Autodesk Fusion 360 part; units mm, degrees
(part 12 of 25)
  arc A2061 (18.3325, 43.4756) -> (18.0149, 43.4756) centre (18.1737, 43.4756) ccw
  arc A2062 (27.9971, 41.2945) -> (28.3146, 41.2945) centre (28.1559, 41.2945) ccw
  arc A2063 (24.9949, 41.4591) -> (24.9949, 41.7766) centre (24.9949, 41.6179) ccw
  arc A2064 (4.8319, 35.4266) -> (4.8319, 35.1091) centre (4.8319, 35.2678) ccw
  arc A2065 (18.3765, 38.645) -> (18.6594, 38.5008) centre (18.5179, 38.5729) ccw
  line L663 (18.8179, 41.8997) -> (18.3999, 41.4817)
  arc A2066 (18.7474, 38.6736) -> (18.4645, 38.8177) centre (18.606, 38.7457) ccw
  line L664 (18.458, 38.3885) -> (18.4277, 38.197)
  line L665 (21.7972, 41.91) -> (21.8221, 41.9203)
  arc A2067 (22.1278, 43.9094) -> (22.3523, 44.1339) centre (22.2401, 44.0217) ccw
  arc A2068 (27.2855, 43.2371) -> (27.2855, 43.5546) centre (27.2855, 43.3959) ccw
  arc A2069 (18.5865, 38.197) -> (18.269, 38.197) centre (18.4277, 38.197) ccw
  arc A2070 (27.3977, 43.5082) -> (27.1732, 43.2836) centre (27.2855, 43.3959) ccw
  arc A2071 (18.5122, 42.4506) -> (18.2877, 42.226) centre (18.4, 42.3383) ccw
  line L666 (18.4277, 38.197) -> (18.4277, 38.1)
  line L667 (21.8221, 41.9203) -> (22.2401, 42.3383)
  arc A2072 (19.1107, 39.0872) -> (19.2322, 39.3805) centre (19.1715, 39.2339) ccw
  line L668 (26.0545, 43.3959) -> (25.1841, 42.5255)
  arc A2073 (18.3204, 42.9452) -> (18.027, 42.8237) centre (18.1737, 42.8845) ccw
  arc A2074 (24.8827, 41.7302) -> (25.1072, 41.5056) centre (24.9949, 41.6179) ccw
  line L669 (18.8571, 39.0396) -> (18.72, 38.9025)
  arc A2075 (18.8786, 42.067) -> (18.7572, 41.7736) centre (18.8179, 41.9203) ccw
  line L670 (28.1559, 41.2945) -> (28.1559, 42.5255)
  line L671 (19.364, 44.6659) -> (18.8179, 44.4397)
  arc A2076 (26.0545, 43.5546) -> (26.0545, 43.2371) centre (26.0545, 43.3959) ccw
  line L672 (22.2401, 42.3383) -> (22.4663, 42.8844)
  arc A2077 (22.625, 43.4756) -> (22.3075, 43.4756) centre (22.4663, 43.4756) ccw
  arc A2078 (26.1668, 43.2836) -> (25.9423, 43.5082) centre (26.0545, 43.3959) ccw
  arc A2079 (18.2877, 44.1339) -> (18.5122, 43.9094) centre (18.4, 44.0217) ccw
  line L673 (18.518, 38.5729) -> (18.458, 38.3885)
  line L674 (18.1737, 40.9356) -> (18.1737, 40.3444)
  arc A2080 (21.8579, 42.0567) -> (21.7364, 41.7633) centre (21.7972, 41.91) ccw
  arc A2081 (18.269, 38.1) -> (18.5865, 38.1) centre (18.4277, 38.1) ccw
  line L675 (22.4663, 43.4756) -> (22.2401, 44.0217)
  arc A2082 (25.2964, 41.6948) -> (25.0718, 41.9193) centre (25.1841, 41.807) ccw
  arc A2083 (18.027, 43.5363) -> (18.3204, 43.4148) centre (18.1737, 43.4755) ccw
  arc A2084 (18.027, 40.9963) -> (18.3204, 40.8748) centre (18.1737, 40.9356) ccw
  arc A2085 (18.4776, 38.839) -> (18.7344, 38.6523) centre (18.606, 38.7456) ccw
  arc A2086 (18.3071, 38.4375) -> (18.609, 38.3394) centre (18.4581, 38.3885) ccw
  arc A2087 (18.2532, 42.2776) -> (18.5466, 42.3991) centre (18.3999, 42.3383) ccw
  line L676 (21.4533, 36.9584) -> (21.6261, 37.0464)
  arc A2088 (18.2709, 38.2218) -> (18.5845, 38.1721) centre (18.4277, 38.197) ccw
  arc A2089 (19.4248, 44.5192) -> (19.3033, 44.8126) centre (19.364, 44.6659) ccw
  line L677 (19.0139, 39.1536) -> (18.8571, 39.0396)
  arc A2090 (18.6689, 38.5238) -> (18.367, 38.6219) centre (18.518, 38.5729) ccw
  arc A2091 (18.7821, 41.7633) -> (18.9035, 42.0567) centre (18.8428, 41.91) ccw
  arc A2092 (18.3204, 40.4052) -> (18.027, 40.2837) centre (18.1737, 40.3444) ccw
  arc A2093 (19.2435, 39.0924) -> (19.0994, 39.3753) centre (19.1715, 39.2339) ccw
  arc A2094 (18.9302, 41.7874) -> (18.7056, 42.0119) centre (18.8179, 41.8997) ccw
  line L678 (18.606, 38.7457) -> (18.518, 38.5729)
  line L679 (18.8179, 39.3803) -> (19.1715, 39.2339)
  arc A2095 (18.7638, 39.1681) -> (18.9504, 38.9112) centre (18.8571, 39.0397) ccw
  arc A2096 (18.9036, 41.7633) -> (18.7821, 42.0567) centre (18.8429, 41.91) ccw
  line L680 (19.1715, 39.2339) -> (19.0139, 39.1536)
  arc A2097 (18.3325, 40.9356) -> (18.0149, 40.9356) centre (18.1737, 40.9356) ccw
  arc A2098 (18.5466, 43.9609) -> (18.2532, 44.0824) centre (18.3999, 44.0217) ccw
  line L681 (18.3999, 42.3383) -> (18.8179, 41.9203)
  line L682 (18.1737, 40.3444) -> (18.3999, 39.7983)
  arc A2099 (18.7056, 41.8081) -> (18.9302, 42.0326) centre (18.8179, 41.9203) ccw
  arc A2100 (18.0149, 40.3444) -> (18.3325, 40.3444) centre (18.1737, 40.3444) ccw
  line L683 (18.3999, 44.0217) -> (18.1737, 43.4756)
  line L684 (18.3999, 39.7983) -> (18.8179, 39.3803)
  arc A2101 (18.9419, 39.2951) -> (19.086, 39.0122) centre (19.014, 39.1537) ccw
  arc A2102 (19.1073, 39.0252) -> (18.9206, 39.282) centre (19.014, 39.1536) ccw
  arc A2103 (18.8484, 38.8092) -> (18.5915, 38.9958) centre (18.72, 38.9025) ccw
  line L685 (18.1737, 43.4756) -> (18.1737, 42.8844)
  arc A2104 (18.7056, 39.2681) -> (18.9302, 39.4926) centre (18.8179, 39.3803) ccw
  arc A2105 (18.2532, 39.7376) -> (18.5466, 39.8591) centre (18.3999, 39.7984) ccw
  line L686 (18.8179, 41.9203) -> (18.8428, 41.91)
  line L687 (18.72, 38.9025) -> (18.606, 38.7457)
  line L688 (18.3999, 41.4817) -> (18.1737, 40.9356)
  line L689 (18.8428, 41.91) -> (18.8179, 41.8997)
  line L690 (18.8179, 44.4397) -> (18.3999, 44.0217)
  arc A2106 (21.2937, 36.7416) -> (21.244, 37.0552) centre (21.2689, 36.8984) ccw
  arc A2107 (18.7572, 42.0463) -> (18.8787, 41.753) centre (18.818, 41.8997) ccw
  arc A2108 (18.8787, 39.527) -> (18.7572, 39.2336) centre (18.8179, 39.3803) ccw
  arc A2109 (18.9693, 38.9274) -> (18.7448, 39.1519) centre (18.8571, 39.0397) ccw
  arc A2110 (18.0149, 42.8844) -> (18.3325, 42.8844) centre (18.1737, 42.8844) ccw
  arc A2111 (18.5122, 39.9106) -> (18.2877, 39.686) centre (18.4, 39.7983) ccw
  arc A2112 (18.6077, 39.0148) -> (18.8322, 38.7903) centre (18.72, 38.9026) ccw
  arc A2113 (18.6148, 38.3636) -> (18.3012, 38.4133) centre (18.458, 38.3884) ccw
  line L691 (18.1737, 42.8844) -> (18.3999, 42.3383)
  arc A2114 (18.2877, 41.5939) -> (18.5122, 41.3694) centre (18.4, 41.4817) ccw
  arc A2115 (33.9077, 4.9657) -> (34.1322, 4.7412) centre (34.02, 4.8535) ccw
  arc A2116 (21.1166, 13.6842) -> (21.1166, 14.0017) centre (21.1166, 13.843) ccw
  arc A2117 (13.9383, 12.0328) -> (13.6208, 12.0328) centre (13.7796, 12.0328) ccw
  line L692 (33.3711, 4.5847) -> (34.02, 4.8535)
  arc A2118 (13.8918, 10.9141) -> (13.6672, 10.6896) centre (13.7795, 10.8018) ccw
  arc A2119 (34.4478, 4.7412) -> (34.6723, 4.9657) centre (34.5601, 4.8535) ccw
  arc A2120 (35.2089, 4.7435) -> (35.2089, 4.426) centre (35.2089, 4.5848) ccw
  arc A2121 (16.3207, 14.0017) -> (16.3207, 13.6842) centre (16.3207, 13.843) ccw
  line L693 (31.6665, 5.207) -> (32.02, 4.8535)
  arc A2122 (17.1338, 11.4447) -> (16.9093, 11.6693) centre (17.0216, 11.557) ccw
  line L694 (22.559, 12.0525) -> (22.86, 12.3536)
  line L695 (16.3207, 13.843) -> (15.9006, 13.669)
  arc A2123 (16.639, 11.399) -> (16.8636, 11.1745) centre (16.7513, 11.2867) ccw
  line L696 (15.8809, 9.9314) -> (16.7513, 10.8018)
  arc A2124 (21.8174, 11.3983) -> (21.8174, 11.7157) centre (21.8174, 11.557) ccw
  arc A2125 (15.7686, 10.0437) -> (15.9931, 9.8191) centre (15.8808, 9.9314) ccw
  line L697 (34.29, 5.1235) -> (34.56, 4.8535)
  arc A2126 (22.9723, 12.4658) -> (22.7477, 12.2413) centre (22.86, 12.3536) ccw
  arc A2127 (16.8636, 10.6896) -> (16.639, 10.9141) centre (16.7513, 10.8019) ccw
  arc A2128 (22.2982, 11.5843) -> (22.1767, 11.8777) centre (22.2375, 11.731) ccw
  line L698 (13.7795, 10.8018) -> (14.6499, 9.9314)
  arc A2129 (35.1481, 4.438) -> (35.2696, 4.7314) centre (35.2088, 4.5847) ccw
  line L699 (16.7513, 11.2868) -> (17.0215, 11.557)
  arc A2130 (31.6665, 5.0482) -> (31.6665, 5.3658) centre (31.6665, 5.207) ccw
  line L700 (14.6499, 9.9314) -> (15.8809, 9.9314)
  arc A2131 (32.6081, 4.438) -> (32.7296, 4.7314) centre (32.6689, 4.5847) ccw
  line L701 (16.7513, 10.8018) -> (16.7513, 11.2868)
  arc A2132 (15.8809, 9.7727) -> (15.8809, 10.0901) centre (15.8809, 9.9314) ccw
  arc A2133 (21.7566, 11.7037) -> (21.8781, 11.4103) centre (21.8173, 11.557) ccw
  arc A2134 (16.91, 11.2868) -> (16.5925, 11.2868) centre (16.7513, 11.2868) ccw
  line L702 (29.8325, 5.381) -> (30.2526, 5.207)
  line L703 (35.2089, 4.5847) -> (35.9111, 4.5847)
  arc A2135 (29.7203, 5.2688) -> (29.9448, 5.4933) centre (29.8326, 5.3811) ccw
  arc A2136 (34.0807, 4.7068) -> (33.9592, 5.0001) centre (34.02, 4.8535) ccw
  arc A2137 (30.1919, 5.0603) -> (30.3134, 5.3537) centre (30.2527, 5.207) ccw
  line L704 (30.2526, 5.207) -> (31.6665, 5.207)
  arc A2138 (14.5377, 9.8191) -> (14.7622, 10.0437) centre (14.65, 9.9314) ccw
  arc A2139 (16.5925, 10.8018) -> (16.91, 10.8018) centre (16.7513, 10.8018) ccw
  line L705 (21.8174, 11.557) -> (22.2375, 11.731)
  arc A2140 (35.8504, 4.7314) -> (35.9719, 4.438) centre (35.9112, 4.5847) ccw
  arc A2141 (30.2526, 5.3658) -> (30.2526, 5.0482) centre (30.2526, 5.207) ccw
  arc A2142 (22.1252, 11.8433) -> (22.3497, 11.6188) centre (22.2375, 11.731) ccw
  line L706 (32.02, 4.8535) -> (32.6689, 4.5847)
  line L707 (34.56, 4.8535) -> (35.2089, 4.5847)
  arc A2143 (31.9078, 4.7412) -> (32.1323, 4.9657) centre (32.0201, 4.8535) ccw
  arc A2144 (29.8933, 5.5277) -> (29.7718, 5.2343) centre (29.8325, 5.381) ccw
  arc A2145 (36.6207, 4.7068) -> (36.4992, 5.0001) centre (36.56, 4.8534) ccw
  line L708 (22.2375, 11.731) -> (22.559, 12.0525)
  arc A2146 (21.6047, 15.0442) -> (21.8293, 15.2687) centre (21.717, 15.1564) ccw
  arc A2147 (34.4023, 5.0112) -> (34.1777, 5.2357) centre (34.29, 5.1235) ccw
  arc A2148 (32.0808, 5.0001) -> (31.9593, 4.7068) centre (32.0201, 4.8534) ccw
  arc A2149 (31.7787, 5.3193) -> (31.5542, 5.0947) centre (31.6665, 5.207) ccw
  arc A2150 (34.4023, 5.2357) -> (34.1777, 5.0112) centre (34.29, 5.1234) ccw
  line L709 (35.9111, 4.5847) -> (36.56, 4.8535)
  arc A2151 (34.6208, 5.0001) -> (34.4993, 4.7068) centre (34.5601, 4.8535) ccw
  arc A2152 (22.9723, 12.2413) -> (22.7477, 12.4658) centre (22.86, 12.3536) ccw
  line L710 (17.0215, 11.557) -> (21.8174, 11.557)
  arc A2153 (22.4467, 12.1648) -> (22.6712, 11.9403) centre (22.5589, 12.0526) ccw
  arc A2154 (14.6499, 10.0901) -> (14.6499, 9.7727) centre (14.6499, 9.9314) ccw
  line L711 (32.6689, 4.5847) -> (33.3711, 4.5847)
  arc A2155 (35.9111, 4.426) -> (35.9111, 4.7435) centre (35.9111, 4.5848) ccw
  arc A2156 (22.6712, 11.9403) -> (22.4467, 12.1648) centre (22.5589, 12.0526) ccw
  arc A2157 (17.0215, 11.7157) -> (17.0215, 11.3983) centre (17.0215, 11.557) ccw
  line L712 (22.86, 12.3536) -> (29.8325, 5.381)
  arc A2158 (38.1941, 4.9955) -> (38.2438, 4.6819) centre (38.2189, 4.8387) ccw
  line L713 (37.7461, 4.8759) -> (37.9811, 4.8387)
  arc A2159 (38.2588, 6.35) -> (37.9413, 6.35) centre (38.1, 6.35) ccw
  arc A2160 (39.5995, 5.4777) -> (39.375, 5.2532) centre (39.4873, 5.3655) ccw
  arc A2161 (37.5689, 5.1004) -> (37.4708, 4.7984) centre (37.5199, 4.9494) ccw
  arc A2162 (38.6081, 5.0909) -> (38.7522, 4.808) centre (38.6802, 4.9495) ccw
  arc A2163 (37.9412, 4.8387) -> (38.2587, 4.8387) centre (38.0999, 4.8387) ccw
  line L714 (39.4872, 5.3655) -> (39.6555, 5.1972)
  arc A2164 (39.365, 5.2532) -> (39.1405, 5.4777) centre (39.2528, 5.3655) ccw
  line L715 (34.02, 4.8535) -> (34.29, 5.1235)
  arc A2165 (33.3104, 4.7314) -> (33.4319, 4.438) centre (33.3712, 4.5847) ccw
  arc A2166 (38.2189, 4.6799) -> (38.2189, 4.9975) centre (38.2189, 4.8387) ccw
  line L716 (37.1155, 5.1972) -> (37.3079, 5.0574)
  arc A2167 (39.5432, 5.085) -> (39.7677, 5.3095) centre (39.6555, 5.1973) ccw
  arc A2168 (37.9562, 4.6819) -> (38.0059, 4.9955) centre (37.9811, 4.8387) ccw
  arc A2169 (38.1, 6.5087) -> (38.1, 6.1912) centre (38.1, 6.35) ccw
  line L717 (37.9811, 4.8387) -> (38.1, 4.8387)
  arc A2170 (39.9878, 4.808) -> (40.1319, 5.0909) centre (40.0599, 4.9494) ccw
  line L718 (38.1, 4.8387) -> (38.2189, 4.8387)
  line L719 (39.6555, 5.1972) -> (39.8479, 5.0574)
  line L720 (38.1, 4.8387) -> (38.1, 6.35)
  line L721 (37.0096, 5.3031) -> (37.1155, 5.1972)
  line L722 (39.37, 5.5268) -> (39.4872, 5.3655)
  arc A2171 (38.4048, 5.0269) -> (38.503, 4.7249) centre (38.4539, 4.8759) ccw
  arc A2172 (38.9642, 4.916) -> (38.82, 5.1989) centre (38.8921, 5.0575) ccw
  line L723 (38.6801, 4.9494) -> (38.8921, 5.0574)
  line L724 (38.8921, 5.0574) -> (39.0845, 5.1972)
  arc A2173 (39.7488, 5.3257) -> (39.5621, 5.0688) centre (39.6555, 5.1973) ccw
  arc A2174 (37.7709, 5.0327) -> (37.7213, 4.7191) centre (37.7461, 4.8759) ccw
  arc A2175 (37.1219, 5.1908) -> (36.8973, 5.4153) centre (37.0096, 5.3031) ccw
  line L725 (37.3079, 5.0574) -> (37.5199, 4.9494)
  arc A2176 (37.0032, 5.085) -> (37.2277, 5.3095) centre (37.1155, 5.1973) ccw
  line L726 (37.5199, 4.9494) -> (37.7461, 4.8759)
  line L727 (39.8479, 5.0574) -> (40.0599, 4.9494)
  arc A2177 (37.9413, 4.8387) -> (38.2588, 4.8387) centre (38.1, 4.8387) ccw
  arc A2178 (38.7292, 4.7984) -> (38.6311, 5.1004) centre (38.6802, 4.9494) ccw
  arc A2179 (38.1, 4.6799) -> (38.1, 4.9974) centre (38.1, 4.8387) ccw
  arc A2180 (38.9723, 5.3095) -> (39.1968, 5.085) centre (39.0846, 5.1973) ccw
  arc A2181 (38.1, 6.1912) -> (38.1, 6.5087) centre (38.1, 6.35) ccw
  line L728 (40.0599, 4.9494) -> (40.2861, 4.8759)
  arc A2182 (33.3711, 4.426) -> (33.3711, 4.7435) centre (33.3711, 4.5848) ccw
  arc A2183 (38.2587, 6.35) -> (37.9412, 6.35) centre (38.0999, 6.35) ccw
  line L729 (38.4539, 4.8759) -> (38.6801, 4.9494)
  arc A2184 (37.9811, 4.9974) -> (37.9811, 4.68) centre (37.9811, 4.8387) ccw
  arc A2185 (39.7546, 4.929) -> (39.9412, 5.1858) centre (39.8479, 5.0574) ccw
  line L730 (39.2528, 5.3655) -> (39.37, 5.5268)
  arc A2186 (38.4787, 4.7191) -> (38.4291, 5.0327) centre (38.4539, 4.8759) ccw
  arc A2187 (38.7988, 5.1858) -> (38.9854, 4.929) centre (38.8921, 5.0574) ccw
  arc A2188 (39.92, 5.1989) -> (39.7758, 4.916) centre (39.8479, 5.0574) ccw
  arc A2189 (40.237, 4.7249) -> (40.3352, 5.0269) centre (40.2861, 4.8759) ccw
  arc A2190 (39.3588, 5.2721) -> (39.6157, 5.4588) centre (39.4873, 5.3654) ccw
  line L731 (39.0845, 5.1972) -> (39.2528, 5.3655)
  line L732 (36.56, 4.8535) -> (37.0096, 5.3031)
  line L733 (38.1, 6.35) -> (38.1, 4.8387)
  arc A2191 (37.4478, 4.808) -> (37.5919, 5.0909) centre (37.5199, 4.9494) ccw
  arc A2192 (38.1, 4.9975) -> (38.1, 4.6799) centre (38.1, 4.8387) ccw
  arc A2193 (36.4477, 4.9657) -> (36.6722, 4.7412) centre (36.56, 4.8535) ccw
  arc A2194 (39.1243, 5.4588) -> (39.3812, 5.2721) centre (39.2527, 5.3655) ccw
  arc A2195 (32.6689, 4.7435) -> (32.6689, 4.426) centre (32.6689, 4.5848) ccw
  arc A2196 (37.38, 5.1989) -> (37.2358, 4.916) centre (37.3079, 5.0575) ccw
  arc A2197 (37.1219, 5.4153) -> (36.8973, 5.1908) centre (37.0096, 5.303) ccw
  arc A2198 (39.4984, 5.4335) -> (39.2416, 5.6201) centre (39.37, 5.5268) ccw
  arc A2199 (39.4984, 5.6201) -> (39.2416, 5.4335) centre (39.37, 5.5268) ccw
  arc A2200 (37.697, 4.7249) -> (37.7952, 5.0269) centre (37.7461, 4.8759) ccw
  arc A2201 (45.3689, 4.7435) -> (45.3689, 4.426) centre (45.3689, 4.5848) ccw
  line L734 (46.72, 4.8535) -> (46.99, 5.1235)
  line L735 (41.6245, 5.1972) -> (41.7304, 5.3031)
  line L736 (46.99, 5.1235) -> (47.26, 4.8535)
  arc A2202 (46.0711, 4.426) -> (46.0711, 4.7435) centre (46.0711, 4.5848) ccw
  arc A2203 (37.2088, 5.3257) -> (37.0221, 5.0688) centre (37.1155, 5.1973) ccw
  arc A2204 (40.7987, 6.35) -> (40.4812, 6.35) centre (40.6399, 6.35) ccw
  arc A2205 (40.3109, 5.0327) -> (40.2613, 4.7191) centre (40.2861, 4.8759) ccw
  arc A2206 (43.5311, 4.426) -> (43.5311, 4.7435) centre (43.5311, 4.5848) ccw
  arc A2207 (46.0104, 4.7314) -> (46.1319, 4.438) centre (46.0712, 4.5847) ccw
  arc A2208 (41.8426, 5.1908) -> (41.6181, 5.4153) centre (41.7304, 5.3031) ccw
  arc A2209 (40.9448, 5.0269) -> (41.043, 4.7249) centre (40.9939, 4.8759) ccw
  line L737 (43.5311, 4.5847) -> (44.18, 4.8535)
  arc A2210 (40.64, 6.1912) -> (40.64, 6.5087) centre (40.64, 6.35) ccw
  line L738 (44.18, 4.8535) -> (44.45, 5.1235)
  arc A2211 (41.2692, 4.7984) -> (41.1711, 5.1004) centre (41.2202, 4.9494) ccw
  arc A2212 (43.4704, 4.7314) -> (43.5919, 4.438) centre (43.5312, 4.5847) ccw
  arc A2213 (37.2146, 4.929) -> (37.4012, 5.1858) centre (37.3079, 5.0574) ccw
  arc A2214 (41.0187, 4.7191) -> (40.9691, 5.0327) centre (40.9939, 4.8759) ccw
  arc A2215 (40.7589, 4.6799) -> (40.7589, 4.9975) centre (40.7589, 4.8387) ccw
  arc A2216 (41.8426, 5.4153) -> (41.6181, 5.1908) centre (41.7304, 5.303) ccw
  line L739 (40.64, 6.35) -> (40.64, 4.8387)
  arc A2217 (40.64, 6.5087) -> (40.64, 6.1912) centre (40.64, 6.35) ccw
  arc A2218 (40.5211, 4.9974) -> (40.5211, 4.68) centre (40.5211, 4.8387) ccw
  arc A2219 (40.7341, 4.9955) -> (40.7838, 4.6819) centre (40.7589, 4.8387) ccw
  arc A2220 (42.0678, 4.7412) -> (42.2923, 4.9657) centre (42.18, 4.8535) ccw
  arc A2221 (39.1779, 5.0688) -> (38.9912, 5.3257) centre (39.0846, 5.1973) ccw
  arc A2222 (46.6077, 4.9657) -> (46.8322, 4.7412) centre (46.72, 4.8534) ccw
  line L740 (42.18, 4.8535) -> (42.8289, 4.5847)
  line L741 (41.4321, 5.0574) -> (41.6245, 5.1972)
  arc A2223 (44.0677, 4.9657) -> (44.2922, 4.7412) centre (44.18, 4.8535) ccw
  line L742 (44.72, 4.8535) -> (45.3689, 4.5847)
  arc A2224 (41.5042, 4.916) -> (41.36, 5.1989) centre (41.4321, 5.0575) ccw
  arc A2225 (41.7179, 5.0688) -> (41.5312, 5.3257) centre (41.6246, 5.1973) ccw
  arc A2226 (40.64, 4.6799) -> (40.64, 4.9974) centre (40.64, 4.8387) ccw
  line L743 (41.2201, 4.9494) -> (41.4321, 5.0574)
  arc A2227 (42.8289, 4.7435) -> (42.8289, 4.426) centre (42.8289, 4.5848) ccw
  arc A2228 (40.4813, 4.8387) -> (40.7988, 4.8387) centre (40.6401, 4.8387) ccw
  line L744 (44.45, 5.1235) -> (44.72, 4.8535)
  line L745 (38.2189, 4.8387) -> (38.4539, 4.8759)
  line L746 (45.3689, 4.5847) -> (46.0711, 4.5847)
  line L747 (41.7304, 5.3031) -> (42.18, 4.8535)
  arc A2229 (47.1023, 5.0112) -> (46.8777, 5.2357) centre (46.99, 5.1234) ccw
  arc A2230 (44.5623, 5.0112) -> (44.3377, 5.2357) centre (44.45, 5.1234) ccw
  arc A2231 (42.2408, 5.0001) -> (42.1193, 4.7068) centre (42.18, 4.8535) ccw
  arc A2232 (44.2407, 4.7068) -> (44.1192, 5.0001) centre (44.18, 4.8534) ccw
  arc A2233 (41.1481, 5.0909) -> (41.2922, 4.808) centre (41.2202, 4.9494) ccw
  arc A2234 (42.7681, 4.438) -> (42.8896, 4.7314) centre (42.8289, 4.5847) ccw
  line L748 (40.9939, 4.8759) -> (41.2201, 4.9494)
  arc A2235 (40.7988, 6.35) -> (40.4813, 6.35) centre (40.6401, 6.35) ccw
  arc A2236 (46.7807, 4.7068) -> (46.6592, 5.0001) centre (46.7199, 4.8535) ccw
  arc A2237 (41.5123, 5.3095) -> (41.7368, 5.085) centre (41.6246, 5.1973) ccw
  line L749 (42.8289, 4.5847) -> (43.5311, 4.5847)
  arc A2238 (44.6078, 4.7412) -> (44.8323, 4.9657) centre (44.72, 4.8535) ccw
  arc A2239 (40.4962, 4.6819) -> (40.5459, 4.9955) centre (40.5211, 4.8387) ccw
  line L750 (40.2861, 4.8759) -> (40.5211, 4.8387)
  line L751 (46.0711, 4.5847) -> (46.72, 4.8535)
  arc A2240 (44.5623, 5.2357) -> (44.3377, 5.0112) centre (44.45, 5.1234) ccw
  line L752 (40.64, 4.8387) -> (40.7589, 4.8387)
  arc A2241 (40.4812, 4.8387) -> (40.7987, 4.8387) centre (40.6399, 4.8387) ccw
  line L753 (40.64, 4.8387) -> (40.64, 6.35)
  line L754 (40.7589, 4.8387) -> (40.9939, 4.8759)
  line L755 (40.5211, 4.8387) -> (40.64, 4.8387)
  arc A2242 (41.3388, 5.1858) -> (41.5254, 4.929) centre (41.4321, 5.0574) ccw
  line L756 (57.15, 5.1235) -> (57.42, 4.8535)
  arc A2243 (49.3207, 4.7068) -> (49.1992, 5.0001) centre (49.26, 4.8535) ccw
  arc A2244 (51.1511, 4.426) -> (51.1511, 4.7435) centre (51.1511, 4.5848) ccw
  arc A2245 (52.2278, 4.7412) -> (52.4523, 4.9657) centre (52.34, 4.8535) ccw
  line L757 (51.8, 4.8535) -> (52.07, 5.1235)
  line L758 (49.53, 5.1235) -> (49.8, 4.8535)
  arc A2246 (52.4008, 5.0001) -> (52.2793, 4.7068) centre (52.34, 4.8535) ccw
  line L759 (53.6911, 4.5847) -> (54.34, 4.8535)
  arc A2247 (49.1477, 4.9657) -> (49.3722, 4.7412) centre (49.26, 4.8535) ccw
  arc A2248 (51.6877, 4.9657) -> (51.9122, 4.7412) centre (51.7999, 4.8535) ccw
  line L760 (54.88, 4.8535) -> (55.5289, 4.5847)
  line L761 (50.4489, 4.5847) -> (51.1511, 4.5847)
  arc A2249 (40.64, 4.9975) -> (40.64, 4.6799) centre (40.64, 4.8387) ccw
  arc A2250 (45.3081, 4.438) -> (45.4296, 4.7314) centre (45.3688, 4.5847) ccw
  arc A2251 (54.7223, 5.2357) -> (54.4977, 5.0112) centre (54.61, 5.1234) ccw
  arc A2252 (56.9407, 4.7068) -> (56.8192, 5.0001) centre (56.88, 4.8535) ccw
  arc A2253 (58.0081, 4.438) -> (58.1296, 4.7314) centre (58.0689, 4.5847) ccw
  arc A2254 (44.7808, 5.0001) -> (44.6593, 4.7068) centre (44.7201, 4.8535) ccw
  arc A2255 (40.1089, 5.1004) -> (40.0108, 4.7984) centre (40.0599, 4.9494) ccw
  line L762 (52.07, 5.1235) -> (52.34, 4.8535)
  line L763 (52.34, 4.8535) -> (52.9889, 4.5847)
  arc A2256 (49.6878, 4.7412) -> (49.9123, 4.9657) centre (49.8, 4.8535) ccw
  arc A2257 (47.8481, 4.438) -> (47.9696, 4.7314) centre (47.9089, 4.5847) ccw
  arc A2258 (55.4681, 4.438) -> (55.5896, 4.7314) centre (55.5288, 4.5847) ccw
  arc A2259 (47.9089, 4.7435) -> (47.9089, 4.426) centre (47.9089, 4.5848) ccw
  arc A2260 (47.1478, 4.7412) -> (47.3723, 4.9657) centre (47.2601, 4.8534) ccw
  arc A2261 (57.2623, 5.0112) -> (57.0377, 5.2357) centre (57.15, 5.1234) ccw
  arc A2262 (57.3078, 4.7412) -> (57.5323, 4.9657) centre (57.4201, 4.8534) ccw
  arc A2263 (57.2623, 5.2357) -> (57.0377, 5.0112) centre (57.15, 5.1234) ccw
  line L764 (57.42, 4.8535) -> (58.0689, 4.5847)
  arc A2264 (49.6423, 5.0112) -> (49.4177, 5.2357) centre (49.53, 5.1234) ccw
  arc A2265 (49.6423, 5.2357) -> (49.4177, 5.0112) centre (49.53, 5.1234) ccw
  line L765 (52.9889, 4.5847) -> (53.6911, 4.5847)
  arc A2266 (52.9889, 4.7435) -> (52.9889, 4.426) centre (52.9889, 4.5848) ccw
  line L766 (54.34, 4.8535) -> (54.61, 5.1235)
  arc A2267 (53.6911, 4.426) -> (53.6911, 4.7435) centre (53.6911, 4.5848) ccw
  arc A2268 (48.5504, 4.7314) -> (48.6719, 4.438) centre (48.6112, 4.5847) ccw
  arc A2269 (56.1704, 4.7314) -> (56.2919, 4.438) centre (56.2311, 4.5847) ccw
  line L767 (48.6111, 4.5847) -> (49.26, 4.8535)
  arc A2270 (52.1823, 5.0112) -> (51.9577, 5.2357) centre (52.07, 5.1234) ccw
  arc A2271 (56.2311, 4.426) -> (56.2311, 4.7435) centre (56.2311, 4.5848) ccw
  arc A2272 (56.7677, 4.9657) -> (56.9922, 4.7412) centre (56.88, 4.8534) ccw
  line L768 (55.5289, 4.5847) -> (56.2311, 4.5847)
  line L769 (51.1511, 4.5847) -> (51.8, 4.8535)
  arc A2273 (50.4489, 4.7435) -> (50.4489, 4.426) centre (50.4489, 4.5848) ccw
  line L770 (56.88, 4.8535) -> (57.15, 5.1235)
  arc A2274 (53.6304, 4.7314) -> (53.7519, 4.438) centre (53.6912, 4.5847) ccw
  line L771 (49.26, 4.8535) -> (49.53, 5.1235)
  arc A2275 (49.8608, 5.0001) -> (49.7393, 4.7068) centre (49.8, 4.8535) ccw
  arc A2276 (51.8607, 4.7068) -> (51.7392, 5.0001) centre (51.7999, 4.8534) ccw
  arc A2277 (54.7223, 5.0112) -> (54.4977, 5.2357) centre (54.61, 5.1234) ccw
  arc A2278 (47.3208, 5.0001) -> (47.1993, 4.7068) centre (47.2601, 4.8534) ccw
  arc A2279 (54.2277, 4.9657) -> (54.4522, 4.7412) centre (54.3399, 4.8535) ccw
  arc A2280 (55.5289, 4.7435) -> (55.5289, 4.426) centre (55.5289, 4.5848) ccw
  arc A2281 (50.3881, 4.438) -> (50.5096, 4.7314) centre (50.4489, 4.5847) ccw
  arc A2282 (54.9408, 5.0001) -> (54.8193, 4.7068) centre (54.8801, 4.8535) ccw
  line L772 (56.2311, 4.5847) -> (56.88, 4.8535)
  arc A2283 (47.1023, 5.2357) -> (46.8777, 5.0112) centre (46.99, 5.1234) ccw
  line L773 (47.9089, 4.5847) -> (48.6111, 4.5847)
  line L774 (49.8, 4.8535) -> (50.4489, 4.5847)
  arc A2284 (51.0904, 4.7314) -> (51.2119, 4.438) centre (51.1512, 4.5847) ccw
  arc A2285 (54.7678, 4.7412) -> (54.9923, 4.9657) centre (54.8801, 4.8534) ccw
  line L775 (47.26, 4.8535) -> (47.9089, 4.5847)
  line L776 (63.8511, 4.5847) -> (64.5, 4.8535)
  arc A2286 (64.8823, 5.2357) -> (64.6577, 5.0112) centre (64.77, 5.1235) ccw
  arc A2287 (61.3111, 4.426) -> (61.3111, 4.7435) centre (61.3111, 4.5848) ccw
  arc A2288 (48.6111, 4.426) -> (48.6111, 4.7435) centre (48.6111, 4.5848) ccw
  arc A2289 (52.9281, 4.438) -> (53.0496, 4.7314) centre (52.9888, 4.5847) ccw
  line L777 (54.61, 5.1235) -> (54.88, 4.8535)
  arc A2290 (59.8023, 5.0112) -> (59.5777, 5.2357) centre (59.69, 5.1234) ccw
  arc A2291 (68.1681, 4.438) -> (68.2896, 4.7314) centre (68.2288, 4.5847) ccw
  line L778 (65.04, 4.8535) -> (65.6889, 4.5847)
  arc A2292 (67.1007, 4.7068) -> (66.9792, 5.0001) centre (67.04, 4.8535) ccw
  arc A2293 (68.2289, 4.7435) -> (68.2289, 4.426) centre (68.2289, 4.5848) ccw
  arc A2294 (62.3423, 5.0112) -> (62.1177, 5.2357) centre (62.23, 5.1234) ccw
  arc A2295 (63.7904, 4.7314) -> (63.9119, 4.438) centre (63.8512, 4.5847) ccw
  line L779 (59.96, 4.8535) -> (60.6089, 4.5847)
  arc A2296 (62.3878, 4.7412) -> (62.6123, 4.9657) centre (62.5001, 4.8535) ccw
  arc A2297 (67.4223, 5.2357) -> (67.1977, 5.0112) centre (67.31, 5.1234) ccw
  arc A2298 (57.4808, 5.0001) -> (57.3593, 4.7068) centre (57.4201, 4.8534) ccw
  arc A2299 (59.8478, 4.7412) -> (60.0723, 4.9657) centre (59.9601, 4.8535) ccw
  arc A2300 (66.3304, 4.7314) -> (66.4519, 4.438) centre (66.3912, 4.5847) ccw
  arc A2301 (64.5607, 4.7068) -> (64.4392, 5.0001) centre (64.4999, 4.8535) ccw
  arc A2302 (61.8477, 4.9657) -> (62.0722, 4.7412) centre (61.9599, 4.8535) ccw
  line L780 (58.0689, 4.5847) -> (58.7711, 4.5847)
  arc A2303 (63.0881, 4.438) -> (63.2096, 4.7314) centre (63.1489, 4.5847) ccw
  line L781 (64.77, 5.1235) -> (65.04, 4.8535)
  arc A2304 (59.3077, 4.9657) -> (59.5322, 4.7412) centre (59.42, 4.8535) ccw
  arc A2305 (59.8023, 5.2357) -> (59.5777, 5.0112) centre (59.69, 5.1234) ccw
  arc A2306 (60.6089, 4.7435) -> (60.6089, 4.426) centre (60.6089, 4.5848) ccw
  arc A2307 (67.4223, 5.0112) -> (67.1977, 5.2357) centre (67.31, 5.1234) ccw
  arc A2308 (62.3423, 5.2357) -> (62.1177, 5.0112) centre (62.23, 5.1234) ccw
  arc A2309 (66.9277, 4.9657) -> (67.1522, 4.7412) centre (67.04, 4.8535) ccw
  arc A2310 (58.7104, 4.7314) -> (58.8319, 4.438) centre (58.7711, 4.5847) ccw
  line L782 (59.69, 5.1235) -> (59.96, 4.8535)
  arc A2311 (64.3877, 4.9657) -> (64.6122, 4.7412) centre (64.5, 4.8535) ccw
  line L783 (65.6889, 4.5847) -> (66.3911, 4.5847)
  line L784 (59.42, 4.8535) -> (59.69, 5.1235)
  arc A2312 (64.9278, 4.7412) -> (65.1523, 4.9657) centre (65.0401, 4.8535) ccw
  line L785 (67.58, 4.8535) -> (68.2289, 4.5847)
  line L786 (63.1489, 4.5847) -> (63.8511, 4.5847)
  arc A2313 (54.4007, 4.7068) -> (54.2792, 5.0001) centre (54.34, 4.8535) ccw
  line L787 (67.04, 4.8535) -> (67.31, 5.1235)
  arc A2314 (59.4807, 4.7068) -> (59.3592, 5.0001) centre (59.42, 4.8535) ccw
  line L788 (58.7711, 4.5847) -> (59.42, 4.8535)
  arc A2315 (62.0207, 4.7068) -> (61.8992, 5.0001) centre (61.96, 4.8534) ccw
  arc A2316 (58.7711, 4.426) -> (58.7711, 4.7435) centre (58.7711, 4.5848) ccw
  line L789 (66.3911, 4.5847) -> (67.04, 4.8535)
  arc A2317 (62.5608, 5.0001) -> (62.4393, 4.7068) centre (62.5001, 4.8535) ccw
  arc A2318 (65.6281, 4.438) -> (65.7496, 4.7314) centre (65.6889, 4.5847) ccw
  arc A2319 (64.8823, 5.0112) -> (64.6577, 5.2357) centre (64.77, 5.1235) ccw
  line L790 (62.23, 5.1235) -> (62.5, 4.8535)
  arc A2320 (63.8511, 4.426) -> (63.8511, 4.7435) centre (63.8511, 4.5848) ccw
  arc A2321 (65.6889, 4.7435) -> (65.6889, 4.426) centre (65.6889, 4.5848) ccw
  arc A2322 (67.6408, 5.0001) -> (67.5193, 4.7068) centre (67.58, 4.8534) ccw
  line L791 (60.6089, 4.5847) -> (61.3111, 4.5847)
  arc A2323 (61.2504, 4.7314) -> (61.3719, 4.438) centre (61.3112, 4.5847) ccw
  arc A2324 (66.3911, 4.426) -> (66.3911, 4.7435) centre (66.3911, 4.5848) ccw
  arc A2325 (65.1008, 5.0001) -> (64.9793, 4.7068) centre (65.0401, 4.8534) ccw
  arc A2326 (68.9311, 4.426) -> (68.9311, 4.7435) centre (68.9311, 4.5848) ccw
  line L792 (67.31, 5.1235) -> (67.58, 4.8535)
  line L793 (64.5, 4.8535) -> (64.77, 5.1235)
  arc A2327 (52.1823, 5.2357) -> (51.9577, 5.0112) centre (52.07, 5.1234) ccw
  line L794 (68.2289, 4.5847) -> (68.9311, 4.5847)
  arc A2328 (60.0208, 5.0001) -> (59.8993, 4.7068) centre (59.9601, 4.8535) ccw
  arc A2329 (64.6577, 7.6888) -> (64.8823, 7.4643) centre (64.77, 7.5766) ccw
  line L795 (70.3453, 5.9989) -> (70.3453, 6.7011)
  arc A2330 (64.6577, 7.4643) -> (64.8823, 7.6888) centre (64.77, 7.5766) ccw
  line L796 (64.5, 7.8465) -> (63.8511, 8.1153)
  line L797 (69.58, 4.8535) -> (70.0765, 5.35)
  arc A2331 (68.9919, 8.262) -> (68.8704, 7.9686) centre (68.9312, 8.1153) ccw
  line L798 (68.2289, 8.1153) -> (67.58, 7.8465)
  arc A2332 (63.8511, 7.9565) -> (63.8511, 8.274) centre (63.8511, 8.1152) ccw
  arc A2333 (67.1977, 7.6888) -> (67.4223, 7.4643) centre (67.31, 7.5766) ccw
  line L799 (61.96, 4.8535) -> (62.23, 5.1235)
  arc A2334 (67.1522, 7.9588) -> (66.9277, 7.7343) centre (67.04, 7.8465) ccw
  arc A2335 (66.9792, 7.6999) -> (67.1007, 7.9932) centre (67.04, 7.8466) ccw
  line L800 (62.5, 4.8535) -> (63.1489, 4.5847)
  arc A2336 (63.9119, 8.262) -> (63.7904, 7.9686) centre (63.8512, 8.1153) ccw
  arc A2337 (67.6923, 7.7343) -> (67.4678, 7.9588) centre (67.58, 7.8465) ccw
  arc A2338 (62.6123, 7.7343) -> (62.3878, 7.9588) centre (62.5001, 7.8466) ccw
  arc A2339 (67.5193, 7.9932) -> (67.6408, 7.6999) centre (67.58, 7.8466) ccw
  arc A2340 (69.9643, 7.2377) -> (70.1888, 7.4622) centre (70.0765, 7.35) ccw
  arc A2341 (70.1888, 5.2378) -> (69.9643, 5.4623) centre (70.0765, 5.3501) ccw
  arc A2342 (66.4519, 8.262) -> (66.3304, 7.9686) centre (66.3912, 8.1153) ccw
  arc A2343 (62.4393, 7.9932) -> (62.5608, 7.6999) centre (62.5001, 7.8466) ccw
  arc A2344 (69.6922, 7.9588) -> (69.4677, 7.7343) centre (69.5799, 7.8465) ccw
  line L801 (68.9311, 4.5847) -> (69.58, 4.8535)
  arc A2345 (63.1489, 4.7435) -> (63.1489, 4.426) centre (63.1489, 4.5848) ccw
  line L802 (62.23, 7.5765) -> (61.96, 7.8465)
  arc A2346 (62.1177, 7.4643) -> (62.3423, 7.6888) centre (62.23, 7.5765) ccw
  arc A2347 (64.6122, 7.9588) -> (64.3877, 7.7343) centre (64.5, 7.8465) ccw
  line L803 (67.58, 7.8465) -> (67.31, 7.5765)
  arc A2348 (63.2096, 7.9686) -> (63.0881, 8.262) centre (63.1489, 8.1153) ccw
  line L804 (69.58, 7.8465) -> (68.9311, 8.1153)
  arc A2349 (70.2232, 7.4107) -> (69.9299, 7.2892) centre (70.0766, 7.35) ccw
  line L805 (63.8511, 8.1153) -> (63.1489, 8.1153)
  line L806 (62.5, 7.8465) -> (62.23, 7.5765)
  arc A2350 (68.9311, 7.9565) -> (68.9311, 8.274) centre (68.9311, 8.1152) ccw
  arc A2351 (62.0722, 7.9588) -> (61.8477, 7.7343) centre (61.9599, 7.8466) ccw
  arc A2352 (68.8704, 4.7314) -> (68.9919, 4.438) centre (68.9312, 4.5847) ccw
  arc A2353 (69.5192, 7.6999) -> (69.6407, 7.9932) centre (69.5799, 7.8465) ccw
  line L807 (67.04, 7.8465) -> (66.3911, 8.1153)
  line L808 (64.77, 7.5765) -> (64.5, 7.8465)
  line L809 (61.96, 7.8465) -> (61.3111, 8.1153)
  line L810 (70.0765, 5.35) -> (70.3453, 5.9989)
  line L811 (61.3111, 4.5847) -> (61.96, 4.8535)
  arc A2354 (70.492, 5.9381) -> (70.1986, 6.0596) centre (70.3453, 5.9989) ccw
  arc A2355 (60.5481, 4.438) -> (60.6696, 4.7314) centre (60.6089, 4.5847) ccw
  line L812 (63.1489, 8.1153) -> (62.5, 7.8465)
  line L813 (68.9311, 8.1153) -> (68.2289, 8.1153)
  arc A2356 (69.9299, 5.4108) -> (70.2232, 5.2893) centre (70.0766, 5.35) ccw
  arc A2357 (67.4678, 4.7412) -> (67.6923, 4.9657) centre (67.58, 4.8534) ccw
  arc A2358 (58.0689, 4.7435) -> (58.0689, 4.426) centre (58.0689, 4.5848) ccw
  line L814 (65.6889, 8.1153) -> (65.04, 7.8465)
  arc A2359 (65.1523, 7.7343) -> (64.9278, 7.9588) centre (65.0401, 7.8465) ccw
  arc A2360 (64.4392, 7.6999) -> (64.5607, 7.9932) centre (64.4999, 7.8466) ccw
  arc A2361 (70.1986, 6.6404) -> (70.492, 6.7619) centre (70.3453, 6.7012) ccw
  arc A2362 (70.504, 6.7011) -> (70.1865, 6.7011) centre (70.3453, 6.7011) ccw
  line L815 (70.3453, 6.7011) -> (70.0765, 7.35)
  arc A2363 (62.1177, 7.6888) -> (62.3423, 7.4643) centre (62.23, 7.5765) ccw
  arc A2364 (63.1489, 8.274) -> (63.1489, 7.9565) centre (63.1489, 8.1152) ccw
  arc A2365 (69.4677, 4.9657) -> (69.6922, 4.7412) centre (69.5799, 4.8534) ccw
  arc A2366 (68.2896, 7.9686) -> (68.1681, 8.262) centre (68.2288, 8.1153) ccw
  arc A2367 (70.1865, 5.9989) -> (70.504, 5.9989) centre (70.3453, 5.9989) ccw
  arc A2368 (68.2289, 8.274) -> (68.2289, 7.9565) centre (68.2289, 8.1152) ccw
  line L816 (57.15, 7.5765) -> (56.88, 7.8465)
  line L817 (52.34, 7.8465) -> (52.07, 7.5765)
  arc A2369 (64.9793, 7.9932) -> (65.1008, 7.6999) centre (65.0401, 7.8466) ccw
  arc A2370 (66.3911, 7.9565) -> (66.3911, 8.274) centre (66.3911, 8.1152) ccw
  line L818 (59.42, 7.8465) -> (58.7711, 8.1153)
  arc A2371 (52.2793, 7.9932) -> (52.4008, 7.6999) centre (52.34, 7.8465) ccw
  arc A2372 (69.6407, 4.7068) -> (69.5192, 5.0001) centre (69.5799, 4.8535) ccw
  arc A2373 (60.6089, 8.274) -> (60.6089, 7.9565) centre (60.6089, 8.1152) ccw
  arc A2374 (51.9577, 7.6888) -> (52.1823, 7.4643) centre (52.07, 7.5765) ccw
  arc A2375 (58.0689, 8.274) -> (58.0689, 7.9565) centre (58.0689, 8.1152) ccw
  arc A2376 (51.9122, 7.9588) -> (51.6877, 7.7343) centre (51.7999, 7.8466) ccw
  arc A2377 (59.5777, 7.4643) -> (59.8023, 7.6888) centre (59.69, 7.5766) ccw
  line L819 (56.2311, 8.1153) -> (55.5289, 8.1153)
  arc A2378 (53.0496, 7.9686) -> (52.9281, 8.262) centre (52.9888, 8.1153) ccw
  arc A2379 (60.0723, 7.7343) -> (59.8478, 7.9588) centre (59.9601, 7.8465) ccw
  arc A2380 (52.4523, 7.7343) -> (52.2278, 7.9588) centre (52.34, 7.8466) ccw
  line L820 (66.3911, 8.1153) -> (65.6889, 8.1153)
  arc A2381 (52.9889, 8.274) -> (52.9889, 7.9565) centre (52.9889, 8.1152) ccw
  line L821 (60.6089, 8.1153) -> (59.96, 7.8465)
  arc A2382 (58.7711, 7.9565) -> (58.7711, 8.274) centre (58.7711, 8.1152) ccw
  line L822 (67.31, 7.5765) -> (67.04, 7.8465)
  line L823 (51.8, 7.8465) -> (51.1511, 8.1153)
  arc A2383 (57.0377, 7.4643) -> (57.2623, 7.6888) centre (57.15, 7.5766) ccw
  line L824 (65.04, 7.8465) -> (64.77, 7.5765)
  arc A2384 (55.5896, 7.9686) -> (55.4681, 8.262) centre (55.5288, 8.1153) ccw
  line L825 (51.1511, 8.1153) -> (50.4489, 8.1153)
  arc A2385 (56.9922, 7.9588) -> (56.7677, 7.7343) centre (56.88, 7.8465) ccw
  arc A2386 (50.4489, 8.274) -> (50.4489, 7.9565) centre (50.4489, 8.1152) ccw
  line L826 (54.88, 7.8465) -> (54.61, 7.5765)
  arc A2387 (54.8193, 7.9932) -> (54.9408, 7.6999) centre (54.8801, 7.8466) ccw
  arc A2388 (65.7496, 7.9686) -> (65.6281, 8.262) centre (65.6889, 8.1153) ccw
  arc A2389 (59.3592, 7.6999) -> (59.4807, 7.9932) centre (59.42, 7.8466) ccw
  arc A2390 (56.2311, 7.9565) -> (56.2311, 8.274) centre (56.2311, 8.1152) ccw
  line L827 (52.9889, 8.1153) -> (52.34, 7.8465)
  arc A2391 (57.0377, 7.6888) -> (57.2623, 7.4643) centre (57.15, 7.5766) ccw
  arc A2392 (61.8992, 7.6999) -> (62.0207, 7.9932) centre (61.9599, 7.8466) ccw
  arc A2393 (51.2119, 8.262) -> (51.0904, 7.9686) centre (51.1512, 8.1153) ccw
  arc A2394 (56.8192, 7.6999) -> (56.9407, 7.9932) centre (56.88, 7.8465) ccw
  arc A2395 (59.5322, 7.9588) -> (59.3077, 7.7343) centre (59.42, 7.8465) ccw
  arc A2396 (57.3593, 7.9932) -> (57.4808, 7.6999) centre (57.4201, 7.8466) ccw
  arc A2397 (58.8319, 8.262) -> (58.7104, 7.9686) centre (58.7711, 8.1153) ccw
  line L828 (54.61, 7.5765) -> (54.34, 7.8465)
  arc A2398 (59.5777, 7.6888) -> (59.8023, 7.4643) centre (59.69, 7.5766) ccw
  arc A2399 (55.5289, 8.274) -> (55.5289, 7.9565) centre (55.5289, 8.1152) ccw
  line L829 (58.7711, 8.1153) -> (58.0689, 8.1153)
  line L830 (59.96, 7.8465) -> (59.69, 7.5765)
  arc A2400 (67.1977, 7.4643) -> (67.4223, 7.6888) centre (67.31, 7.5766) ccw
  arc A2401 (59.8993, 7.9932) -> (60.0208, 7.6999) centre (59.9601, 7.8466) ccw
  line L831 (70.0765, 7.35) -> (69.58, 7.8465)
  arc A2402 (54.4977, 7.6888) -> (54.7223, 7.4643) centre (54.61, 7.5766) ccw
  arc A2403 (51.9577, 7.4643) -> (52.1823, 7.6888) centre (52.07, 7.5765) ccw
  arc A2404 (51.7392, 7.6999) -> (51.8607, 7.9932) centre (51.7999, 7.8466) ccw
  arc A2405 (56.2919, 8.262) -> (56.1704, 7.9686) centre (56.2311, 8.1153) ccw
  line L832 (55.5289, 8.1153) -> (54.88, 7.8465)
  arc A2406 (61.3719, 8.262) -> (61.2504, 7.9686) centre (61.3112, 8.1153) ccw
  arc A2407 (57.5323, 7.7343) -> (57.3078, 7.9588) centre (57.4201, 7.8465) ccw
  arc A2408 (58.1296, 7.9686) -> (58.0081, 8.262) centre (58.0689, 8.1153) ccw
  arc A2409 (54.9923, 7.7343) -> (54.7678, 7.9588) centre (54.8801, 7.8465) ccw
  arc A2410 (65.6889, 8.274) -> (65.6889, 7.9565) centre (65.6889, 8.1152) ccw
  line L833 (52.07, 7.5765) -> (51.8, 7.8465)
  line L834 (58.0689, 8.1153) -> (57.42, 7.8465)
  arc A2411 (56.9749, 34.0406) -> (57.2924, 34.0406) centre (57.1337, 34.0406) ccw
  arc A2412 (56.987, 34.4786) -> (57.2804, 34.6001) centre (57.1337, 34.5394) ccw
  arc A2413 (47.9089, 8.274) -> (47.9089, 7.9565) centre (47.9089, 8.1152) ccw
  line L835 (46.72, 7.8465) -> (46.6979, 7.8557)
  arc A2414 (55.2821, 35.2406) -> (55.0576, 35.4651) centre (55.1698, 35.3528) ccw
  line L836 (46.6979, 13.1749) -> (46.7828, 13.2598)
  line L837 (53.6911, 8.1153) -> (52.9889, 8.1153)
  arc A2415 (61.3111, 7.9565) -> (61.3111, 8.274) centre (61.3111, 8.1152) ccw
  line L838 (49.8, 7.8465) -> (49.53, 7.5765)
  arc A2416 (47.3723, 7.7343) -> (47.1478, 7.9588) centre (47.2601, 7.8465) ccw
  arc A2417 (46.8951, 13.1476) -> (46.6706, 13.3721) centre (46.7829, 13.2599) ccw
  arc A2418 (46.8566, 13.1749) -> (46.5391, 13.1749) centre (46.6979, 13.1749) ccw
  arc A2419 (46.5856, 13.2872) -> (46.8102, 13.0626) centre (46.6979, 13.1749) ccw
  arc A2420 (51.1511, 7.9565) -> (51.1511, 8.274) centre (51.1511, 8.1152) ccw
  line L839 (47.26, 7.8465) -> (46.99, 7.5765)
  arc A2421 (47.1993, 7.9932) -> (47.3208, 7.6999) centre (47.2601, 7.8466) ccw
  arc A2422 (48.6719, 8.262) -> (48.5504, 7.9686) centre (48.6112, 8.1153) ccw
  arc A2423 (49.1992, 7.6999) -> (49.3207, 7.9932) centre (49.26, 7.8466) ccw
  line L840 (49.26, 7.8465) -> (48.6111, 8.1153)
  line L841 (49.53, 7.5765) -> (49.26, 7.8465)
  line L842 (46.6979, 7.8557) -> (46.6979, 13.1749)
  line L843 (46.99, 7.5765) -> (46.72, 7.8465)
  line L844 (50.4489, 8.1153) -> (49.8, 7.8465)
  line L845 (48.6111, 8.1153) -> (47.9089, 8.1153)
  line L846 (57.1337, 34.0406) -> (57.1337, 34.5394)
  line L847 (56.88, 7.8465) -> (56.2311, 8.1153)
  arc A2424 (48.6111, 7.9565) -> (48.6111, 8.274) centre (48.6111, 8.1152) ccw
  arc A2425 (46.8322, 7.9588) -> (46.6077, 7.7343) centre (46.72, 7.8465) ccw
  line L848 (54.6263, 34.5394) -> (54.6263, 34.0406)
  arc A2426 (54.2792, 7.6999) -> (54.4007, 7.9932) centre (54.34, 7.8466) ccw
  arc A2427 (49.4177, 7.6888) -> (49.6423, 7.4643) centre (49.53, 7.5765) ccw
  arc A2428 (60.6696, 7.9686) -> (60.5481, 8.262) centre (60.6089, 8.1153) ccw
  arc A2429 (53.6911, 7.9565) -> (53.6911, 8.274) centre (53.6911, 8.1152) ccw
  arc A2430 (47.9696, 7.9686) -> (47.8481, 8.262) centre (47.9089, 8.1153) ccw
  arc A2431 (54.4796, 34.6001) -> (54.773, 34.4786) centre (54.6263, 34.5393) ccw
  arc A2432 (57.0895, 35.0609) -> (56.7962, 34.9394) centre (56.9429, 35.0001) ccw
  arc A2433 (54.785, 34.5394) -> (54.4676, 34.5394) centre (54.6263, 34.5394) ccw
  line L849 (59.69, 7.5765) -> (59.42, 7.8465)
  arc A2434 (54.4676, 34.0406) -> (54.785, 34.0406) centre (54.6263, 34.0406) ccw
  line L850 (54.8172, 35.0002) -> (54.6263, 34.5394)
  arc A2435 (49.4177, 7.4643) -> (49.6423, 7.6888) centre (49.53, 7.5765) ccw
  arc A2436 (46.8777, 7.6888) -> (47.1023, 7.4643) centre (46.99, 7.5766) ccw
  arc A2437 (54.9638, 34.9394) -> (54.6705, 35.0609) centre (54.8172, 35.0002) ccw
  arc A2438 (46.6592, 7.6999) -> (46.7807, 7.9932) centre (46.7199, 7.8465) ccw
  arc A2439 (50.5096, 7.9686) -> (50.3881, 8.262) centre (50.4489, 8.1153) ccw
  line L851 (61.3111, 8.1153) -> (60.6089, 8.1153)
  line L852 (55.1698, 35.3528) -> (54.8172, 35.0002)
  line L853 (47.9089, 8.1153) -> (47.26, 7.8465)
  arc A2440 (54.4977, 7.4643) -> (54.7223, 7.6888) centre (54.61, 7.5766) ccw
  arc A2441 (53.7519, 8.262) -> (53.6304, 7.9686) centre (53.6912, 8.1153) ccw
  line L854 (57.42, 7.8465) -> (57.15, 7.5765)
  arc A2442 (54.4522, 7.9588) -> (54.2277, 7.7343) centre (54.3399, 7.8466) ccw
  arc A2443 (57.2924, 34.5394) -> (56.9749, 34.5394) centre (57.1337, 34.5394) ccw
  line L855 (56.9428, 35.0002) -> (56.5902, 35.3528)
  line L856 (54.34, 7.8465) -> (53.6911, 8.1153)
  arc A2444 (49.9123, 7.7343) -> (49.6878, 7.9588) centre (49.8, 7.8466) ccw
  arc A2445 (55.6914, 35.397) -> (55.5699, 35.6904) centre (55.6307, 35.5437) ccw
  arc A2446 (49.7393, 7.9932) -> (49.8608, 7.6999) centre (49.8, 7.8466) ccw
  arc A2447 (55.1091, 35.4995) -> (55.2306, 35.2062) centre (55.1698, 35.3529) ccw
  arc A2448 (56.5294, 35.2062) -> (56.6509, 35.4995) centre (56.5902, 35.3529) ccw
  arc A2449 (54.7049, 35.1124) -> (54.9294, 34.8879) centre (54.8172, 35.0002) ccw
  line L857 (68.0202, 17.5728) -> (67.5594, 17.7637)
  arc A2450 (56.8306, 34.8879) -> (57.0551, 35.1124) centre (56.9429, 35.0001) ccw
  arc A2451 (68.7224, 16.7594) -> (68.4049, 16.7594) centre (68.5636, 16.7594) ccw
  arc A2452 (54.9043, 18.4353) -> (55.1976, 18.5568) centre (55.051, 18.496) ccw
  arc A2453 (49.3722, 7.9588) -> (49.1477, 7.7343) centre (49.26, 7.8465) ccw
  arc A2454 (46.6362, 13.3206) -> (46.9295, 13.1991) centre (46.7828, 13.2598) ccw
  line L858 (57.1337, 34.5394) -> (56.9428, 35.0002)
  arc A2455 (56.1901, 35.6904) -> (56.0686, 35.397) centre (56.1294, 35.5437) ccw
  arc A2456 (46.8777, 7.4643) -> (47.1023, 7.6888) centre (46.99, 7.5766) ccw
  arc A2457 (55.6306, 35.7024) -> (55.6306, 35.3849) centre (55.6306, 35.5436) ccw
  line L859 (67.5594, 15.2563) -> (68.0202, 15.4472)
  arc A2458 (67.0606, 17.9224) -> (67.0606, 17.6049) centre (67.0606, 17.7636) ccw
  line L860 (67.0606, 17.7637) -> (66.5998, 17.5728)
  arc A2459 (67.5594, 17.6049) -> (67.5594, 17.9224) centre (67.5594, 17.7636) ccw
  arc A2460 (55.1632, 18.6083) -> (54.9387, 18.3838) centre (55.051, 18.496) ccw
  arc A2461 (67.9079, 15.5594) -> (68.1324, 15.3349) centre (68.0202, 15.4472) ccw
  arc A2462 (67.1214, 17.617) -> (66.9999, 17.9104) centre (67.0606, 17.7637) ccw
  arc A2463 (66.7121, 17.4606) -> (66.4876, 17.6851) centre (66.5999, 17.5728) ccw
  arc A2464 (47.1204, 13.6599) -> (46.827, 13.7814) centre (46.9737, 13.7207) ccw
  line L861 (66.5998, 15.4472) -> (67.0606, 15.2563)
  line L862 (46.7828, 13.2598) -> (46.9737, 13.7206)
  arc A2465 (66.9999, 15.1096) -> (67.1214, 15.403) centre (67.0606, 15.2563) ccw
  line L863 (67.5594, 17.7637) -> (67.0606, 17.7637)
  arc A2466 (68.2262, 15.8606) -> (68.5195, 15.7391) centre (68.3728, 15.7999) ccw
  arc A2467 (54.7898, 33.3826) -> (55.0144, 33.6072) centre (54.9021, 33.4949) ccw
  arc A2468 (68.4851, 15.6876) -> (68.2606, 15.9121) centre (68.3728, 15.7999) ccw
  arc A2469 (57.7032, 16.0683) -> (57.4787, 15.8438) centre (57.591, 15.9561) ccw
  line L864 (66.5149, 17.4879) -> (58.8251, 17.4879)
  arc A2470 (54.9294, 33.6921) -> (54.7049, 33.4676) centre (54.8172, 33.5799) ccw
  line L865 (54.9021, 33.4949) -> (54.9021, 18.8555)
  arc A2471 (46.7586, 8.0024) -> (46.6372, 7.709) centre (46.6979, 7.8557) ccw
  arc A2472 (67.9594, 17.4262) -> (68.0809, 17.7195) centre (68.0202, 17.5728) ccw
  arc A2473 (67.6201, 17.9104) -> (67.4986, 17.617) centre (67.5593, 17.7637) ccw
  line L866 (54.9021, 18.8555) -> (55.051, 18.4961)
  line L867 (55.6306, 35.5437) -> (55.1698, 35.3528)
  line L868 (66.5998, 17.5728) -> (66.5149, 17.4879)
  arc A2474 (57.9268, 15.8276) -> (57.8053, 15.5343) centre (57.8661, 15.6809) ccw
  line L869 (66.5149, 15.5321) -> (66.5998, 15.4472)
  line L870 (56.5902, 35.3528) -> (56.1294, 35.5437)
  line L871 (68.5637, 16.2606) -> (68.5637, 16.7594)
  arc A2475 (54.773, 34.1014) -> (54.4796, 33.9799) centre (54.6263, 34.0406) ccw
  arc A2476 (67.4986, 15.403) -> (67.6201, 15.1096) centre (67.5593, 15.2563) ccw
  arc A2477 (46.5391, 7.8557) -> (46.8566, 7.8557) centre (46.6979, 7.8557) ccw
  arc A2478 (66.5391, 17.7195) -> (66.6606, 17.4262) centre (66.5999, 17.5729) ccw
  line L872 (54.6263, 34.0406) -> (54.8172, 33.5798)
  arc A2479 (68.5195, 17.2809) -> (68.2262, 17.1594) centre (68.3728, 17.2202) ccw
  arc A2480 (68.1324, 17.6851) -> (67.9079, 17.4606) centre (68.0202, 17.5728) ccw
  arc A2481 (54.6705, 33.5191) -> (54.9638, 33.6406) centre (54.8172, 33.5799) ccw
  arc A2482 (68.417, 16.6986) -> (68.7104, 16.8201) centre (68.5637, 16.7594) ccw
  arc A2483 (56.7024, 35.4651) -> (56.4779, 35.2406) centre (56.5902, 35.3529) ccw
  arc A2484 (68.2606, 17.1079) -> (68.4851, 17.3324) centre (68.3728, 17.2202) ccw
  arc A2485 (58.2255, 15.6909) -> (58.2255, 15.3734) centre (58.2255, 15.5321) ccw
  line L873 (56.1294, 35.5437) -> (55.6306, 35.5437)
  arc A2486 (66.4026, 17.6002) -> (66.6272, 17.3756) centre (66.5149, 17.4879) ccw
  arc A2487 (66.6272, 15.6444) -> (66.4026, 15.4198) centre (66.5149, 15.5321) ccw
  arc A2488 (56.1294, 35.3849) -> (56.1294, 35.7024) centre (56.1294, 35.5436) ccw
  line L874 (57.8661, 15.681) -> (58.2255, 15.5321)
  line L875 (68.3728, 17.2202) -> (68.0202, 17.5728)
  arc A2489 (68.5588, 2.0638) -> (68.5588, 1.7463) centre (68.5588, 1.9051) ccw
  arc A2490 (3.696, 3.0163) -> (3.696, 3.3338) centre (3.696, 3.1751) ccw
  arc A2491 (32.964, 1.7463) -> (32.964, 2.0638) centre (32.964, 1.9051) ccw
  line L876 (55.051, 18.4961) -> (57.591, 15.9561)
  arc A2492 (5.0673, 2.6987) -> (5.0673, 2.3813) centre (5.0673, 2.54) ccw
  arc A2493 (66.6606, 15.5938) -> (66.5391, 15.3005) centre (66.5999, 15.4472) ccw
  arc A2494 (57.4787, 15.8438) -> (57.7032, 16.0683) centre (57.591, 15.9561) ccw
  line L877 (68.5637, 16.7594) -> (68.3728, 17.2202)
  arc A2495 (57.7538, 15.5687) -> (57.9783, 15.7932) centre (57.8661, 15.681) ccw
  arc A2496 (73.5277, 1.1113) -> (73.5277, 1.4287) centre (73.5277, 1.27) ccw
  arc A2497 (54.7434, 18.8555) -> (55.0609, 18.8555) centre (54.9021, 18.8555) ccw
  arc A2498 (55.0488, 18.9162) -> (54.7554, 18.7947) centre (54.9021, 18.8555) ccw
  arc A2499 (68.7104, 16.1999) -> (68.417, 16.3214) centre (68.5637, 16.2607) ccw
  arc A2500 (72.4814, 2.3813) -> (72.4814, 2.6987) centre (72.4814, 2.54) ccw
  line L878 (54.8172, 33.5798) -> (54.9021, 33.4949)
  line L879 (58.2255, 15.5321) -> (66.5149, 15.5321)
  arc A2501 (66.5149, 15.3734) -> (66.5149, 15.6909) centre (66.5149, 15.5321) ccw
  arc A2502 (58.8251, 17.6466) -> (58.8251, 17.3291) centre (58.8251, 17.4879) ccw
  arc A2503 (67.5594, 15.0976) -> (67.5594, 15.4151) centre (67.5594, 15.2564) ccw
  line L880 (56.8579, 19.4551) -> (56.8579, 33.4949)
  arc A2504 (5.0673, 2.3813) -> (5.0673, 2.6987) centre (5.0673, 2.54) ccw
  arc A2505 (68.5588, 2.6987) -> (68.5588, 2.3813) centre (68.5588, 2.54) ccw
  arc A2506 (4.331, 2.3813) -> (4.331, 2.6987) centre (4.331, 2.54) ccw
  arc A2507 (6.4386, 3.3338) -> (6.4386, 3.0163) centre (6.4386, 3.1751) ccw
  line L881 (67.0606, 15.2563) -> (67.5594, 15.2563)
  arc A2508 (67.0606, 15.4151) -> (67.0606, 15.0976) centre (67.0606, 15.2564) ccw
  arc A2509 (68.0809, 15.3005) -> (67.9594, 15.5938) centre (68.0202, 15.4472) ccw
  arc A2510 (84.2253, 2.3813) -> (84.2253, 2.6987) centre (84.2253, 2.54) ccw
  arc A2511 (66.4876, 15.3349) -> (66.7121, 15.5594) centre (66.5999, 15.4472) ccw
  arc A2512 (82.5144, 2.6987) -> (82.5144, 2.3813) centre (82.5144, 2.54) ccw
  arc A2513 (0.7747, 3.3338) -> (0.7747, 3.0163) centre (0.7747, 3.1751) ccw
  arc A2514 (58.1647, 15.3854) -> (58.2862, 15.6788) centre (58.2255, 15.5321) ccw
  arc A2515 (55.0609, 33.4949) -> (54.7434, 33.4949) centre (54.9021, 33.4949) ccw
  arc A2516 (12.6114, 3.0163) -> (12.6114, 3.3338) centre (12.6114, 3.1751) ccw
  arc A2517 (13.97, 3.3338) -> (13.97, 3.0163) centre (13.97, 3.1751) ccw
  arc A2518 (56.7456, 33.6072) -> (56.9702, 33.3826) centre (56.8579, 33.4949) ccw
  arc A2519 (68.4049, 16.2606) -> (68.7224, 16.2606) centre (68.5636, 16.2606) ccw
  arc A2520 (56.6991, 19.4551) -> (57.0166, 19.4551) centre (56.8578, 19.4551) ccw
  line L882 (56.9428, 33.5798) -> (57.1337, 34.0406)
  arc A2521 (57.2804, 33.9799) -> (56.987, 34.1014) centre (57.1337, 34.0406) ccw
  arc A2522 (5.0673, 3.3338) -> (5.0673, 3.0163) centre (5.0673, 3.1751) ccw
  arc A2523 (13.97, 3.0163) -> (13.97, 3.3338) centre (13.97, 3.1751) ccw
  line L883 (57.591, 15.9561) -> (57.8661, 15.681)
  arc A2524 (57.0551, 33.4676) -> (56.8306, 33.6921) centre (56.9429, 33.5799) ccw
  line L884 (68.0202, 15.4472) -> (68.3728, 15.7998)
  line L885 (68.3728, 15.7998) -> (68.5637, 16.2606)
  arc A2525 (5.0673, 3.0163) -> (5.0673, 3.3338) centre (5.0673, 3.1751) ccw
  arc A2526 (74.9658, 1.4287) -> (74.9658, 1.1113) centre (74.9658, 1.27) ccw
  arc A2527 (58.7128, 17.3756) -> (58.9373, 17.6002) centre (58.8251, 17.4879) ccw
  line L886 (56.8579, 33.4949) -> (56.9428, 33.5798)
  arc A2528 (40.64, 4.9212) -> (40.64, 5.2388) centre (40.64, 5.08) ccw
  arc A2529 (84.2253, 1.1113) -> (84.2253, 1.4287) centre (84.2253, 1.27) ccw
  arc A2530 (6.4132, 4.6038) -> (6.4132, 4.2862) centre (6.4132, 4.445) ccw
  arc A2531 (81.4682, 1.4287) -> (81.4682, 1.1113) centre (81.4682, 1.27) ccw
  arc A2532 (14.6936, 2.6987) -> (14.6936, 2.3813) centre (14.6936, 2.54) ccw
  arc A2533 (0.7747, 1.4287) -> (0.7747, 1.1113) centre (0.7747, 1.27) ccw
  arc A2534 (0.7747, 2.6987) -> (0.7747, 2.3813) centre (0.7747, 2.54) ccw
  arc A2535 (0.7747, 2.0638) -> (0.7747, 1.7463) centre (0.7747, 1.9051) ccw
  line L887 (58.8251, 17.4879) -> (56.8579, 19.4551)
  arc A2536 (68.5588, 1.4287) -> (68.5588, 1.1113) centre (68.5588, 1.27) ccw
  arc A2537 (33.1022, 3.6513) -> (33.1022, 3.9688) centre (33.1022, 3.81) ccw
  arc A2538 (13.97, 3.9688) -> (13.97, 3.6513) centre (13.97, 3.81) ccw
  arc A2539 (13.2464, 2.3813) -> (13.2464, 2.6987) centre (13.2464, 2.54) ccw
  arc A2540 (82.2548, 2.0638) -> (82.2548, 1.7463) centre (82.2548, 1.9051) ccw
  arc A2541 (41.4632, 5.2388) -> (41.4632, 4.9212) centre (41.4632, 5.08) ccw
  arc A2542 (15.3286, 3.3338) -> (15.3286, 3.0163) centre (15.3286, 3.1751) ccw
  arc A2543 (72.4814, 3.0163) -> (72.4814, 3.3338) centre (72.4814, 3.1751) ccw
  arc A2544 (66.5149, 17.3291) -> (66.5149, 17.6466) centre (66.5149, 17.4879) ccw
  arc A2545 (72.72, 3.6513) -> (72.72, 3.9688) centre (72.72, 3.81) ccw